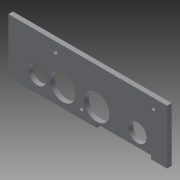
# Autodesk Inventor part: Dish_Injector_Wall
Saved by Autodesk Inventor 2014 (Build 180170000, 170)
## iProperties
Created: 2015-01-07
Part Number: Dish_Injector_Wall
Material: Generic
Document SubType Name: Modeling
Designer: Owner
Density: 1 g/cm^3
Appearance: Default
Author: Owner
Autodesk Inventor part; units mm, degrees
ref_plane "YZ Plane" through (0, 0, 0) normal (1, 0, 0) x (0, 1, 0)
ref_plane "XZ Plane" through (0, 0, 0) normal (0, 1, 0) x (-1, 0, 0)
ref_plane "XY Plane" through (0, 0, 0) normal (0, 0, 1) x (1, 0, 0)
sketch "Sketch1" plane through (0, 0, 0) normal (0, 0, 1) x (1, 0, 0)
  line L0 (-107.2757, 7.2736) -> (3.8493, 7.2736)
  line L1 (3.8493, 7.2736) -> (3.8493, -30.8264)
  line L2 (3.8493, -30.8264) -> (-107.2757, -30.8264)
  line L3 (-107.2757, -30.8264) -> (-107.2757, 7.2736)
  circle A0 centre (-72.1471, 0.8391) radius 1.5875
  circle A1 centre (-53.9997, -24.4192) radius 1.5875
  circle A2 centre (-3.5671, 0.8391) radius 1.5875
  circle A3 centre (-66.6357, -18.1264) radius 8.89
  circle A4 centre (-42.8867, -18.1264) radius 8.89
  circle A5 centre (-81.8757, -19.3964) radius 6.35
  circle A6 centre (-11.1367, -19.3964) radius 6.35
  line L4 (-42.8867, -30.8264) -> (-4.7867, -30.8264)
  line L5 (-4.7867, -30.8264) -> (-4.7867, -28.2864)
  line L6 (-4.7867, -28.2864) -> (-42.8867, -28.2864)
  line L7 (-42.8867, -28.2864) -> (-42.8867, -30.8264)
  line L8 (-46.3681, 7.2736) -> (-20.9681, 7.2736)
  point P0 (0, 0)
  dimension "d2" = 111.125
  dimension "d3" = 38.1
  dimension "d4" = 3.175
  dimension "d5" = 3.175
  dimension "d6" = 3.175
  dimension "d7" = 12.7
  dimension "d8" = 12.7
  dimension "d9" = 17.78
  dimension "d10" = 17.78
  dimension "d11" = 12.7
  dimension "d12" = 12.7
  dimension "d13" = 23.749
  dimension "d14" = 11.43
  dimension "d15" = 11.43
  dimension "d16" = 15.24
  dimension "d17" = 31.75
  dimension "d18" = 6.4345
  dimension "d19" = 6.4345
  dimension "d20" = 68.58
  dimension "d21" = 6.4071
  dimension "d22" = 11.1131
  dimension "d23" = 5.5114
  dimension "d24" = 2.54
  dimension "d25" = 38.1
  dimension "d26" = 0
  dimension "d27" = 25.4
  constraints: 18 end point, 7 centre point, 4 parallel, 3 horizontal, 2 perpendicular, 2 point on line
  measures "d2" distance of L0.start L0.end
  measures "d3" distance of L0.end L1.end
  measures "d4" diameter of A0
  measures "d5" diameter of A2
  measures "d6" diameter of A1
  measures "d7" diameter of A5
  measures "d8" diameter of A6
  measures "d9" diameter of A4
  measures "d10" diameter of A3
  measures "d11" distance from line of L2 A3.centre
  measures "d12" distance from line of L2 A4.centre
  measures "d13" distance of A4.centre A3.centre
  measures "d14" distance from line of L2 A5.centre
  measures "d15" distance from line of L2 A6.centre
  measures "d16" horizontal distance of A3.centre A5.centre
  measures "d17" horizontal distance of A4.centre A6.centre
  measures "d18" distance from line of L0 A0.centre
  measures "d19" distance from line of L0 A2.centre
  measures "d20" distance of A0.centre A2.centre
  measures "d21" distance from line of L2 A1.centre
  measures "d22" horizontal distance of A4.centre A1.centre
  measures "d23" horizontal distance of A0.centre A3.centre
  measures "d24" distance of L4.end L5.end
  measures "d25" distance of L5.end L6.end
  measures "d26" distance from line of A4.centre L7
  measures "d27" distance from line of L3 A5.centre
extrude "Extrusion1" add sketch "Sketch1" along normal blind 3.175 contours L0 L1 L2 L5 L6 L7 L3
body "Solid1"
